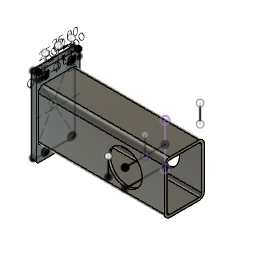
Ensamble-SC280 (Autodesk Fusion 360 archive; units mm, degrees)
design "ApoyoEje1" references "Chasis-V0"
Autodesk Fusion 360 part; units mm, degrees
ref_plane "WorkPlane1" through (506, 300, 480) normal (1, 0, 0) x (0, 1, 0)
sketch "Sketch1" plane through (506, 0, 0) normal (1, 0, 0) x (0, 1, 0)
  line L0 (260, 25) -> (340, 25)
  line L1 (340, 25) -> (340, 935)
  line L2 (340, 935) -> (260, 935)
  line L3 (260, 935) -> (260, 25)
  line L4 (0, 0) -> (600, 0) construction
  line L5 (0, 545) -> (600, 545) construction
  line L6 (328, 595) -> (272, 595)
  line L7 (262, 585) -> (262, 505)
  line L8 (272, 495) -> (328, 495)
  line L9 (338, 505) -> (338, 585)
  arc A0 (338, 585) -> (328, 595) centre (328, 585) ccw
  arc A1 (272, 595) -> (262, 585) centre (272, 585) ccw
  arc A2 (328, 495) -> (338, 505) centre (328, 505) ccw
  arc A3 (262, 505) -> (272, 495) centre (272, 505) ccw
  line L10 (272, 499.8) -> (328, 499.8)
  arc A4 (328, 499.8) -> (333.2, 505) centre (328, 505) ccw
  line L11 (333.2, 505) -> (333.2, 585)
  arc A5 (333.2, 585) -> (328, 590.2) centre (328, 585) ccw
  line L12 (328, 590.2) -> (272, 590.2)
  arc A6 (272, 590.2) -> (266.8, 585) centre (272, 585) ccw
  line L13 (266.8, 585) -> (266.8, 505)
  arc A7 (266.8, 505) -> (272, 499.8) centre (272, 505) ccw
  line L14 (300, 499.8) -> (300, 590.2) construction
  line L15 (333.2, 545) -> (266.8, 545) construction
  line L16 (258.75, 470) -> (341.25, 470)
  point P0 (262, 595)
  point P1 (262, 495)
  point P2 (338, 495)
  point P3 (300, 545)
  point P4 (300, 495)
  point P5 (262, 545)
  point P6 (300, 545)
  point P7 (300, 620)
  dimension "d1" = 76
  dimension "d2" = 100
  dimension "d3" = -4.8
  dimension "d5" = 300
  dimension "d6" = 10
  dimension "d7" = 10
  dimension "d8" = 10
  dimension "d9" = 10
  dimension "d11" = 300
  dimension "d12" = 545
  dimension "d35" = 82.5
  constraint coincident L4.start origin
  constraint horizontal L4
  constraint horizontal L5
  constraint horizontal L6
  constraint perpendicular L6 L7
  constraint parallel L6 L8
  constraint parallel L7 L9
  constraint midpoint L5 P6
  constraint tangent L6 A0
  constraint tangent L9 A0
  constraint coincident P0 L6
  constraint coincident P0 L7
  constraint tangent L6 A1
  constraint tangent L7 A1
  constraint coincident P2 L8
  constraint coincident P2 L9
  constraint tangent L8 A2
  constraint tangent L9 A2
  constraint coincident P1 L7
  constraint coincident P1 L8
  constraint tangent L7 A3
  constraint tangent L8 A3
  constraint midpoint L10 L14.start
  constraint midpoint L12 L14.end
  constraint midpoint L11 L15.start
  constraint midpoint L13 L15.end
  constraint midpoint L8 P4
  constraint midpoint L7 P5
  constraint coincident P6 P3
  measures "d1" distance of P1 P2
  measures "d2" distance of P0 P1
  measures "d5" horizontal distance of L4.start P6
  measures "d6" radius of A0
  measures "d7" radius of A1
  measures "d8" radius of A2
  measures "d9" radius of A3
  measures "d11" horizontal distance of L4.start P4
  measures "d12" vertical distance of L4.start P5
  measures "d35" distance of L16.start L16.end
extrude "Extrude1" add sketch "Sketch1" along normal blind 250 contours L6 L7 L8 L9 A0 A1 A2 A3 makes body 1
extrude "Extrude2" cut 1 faces at (506, 265.2, 558.3333) along direction (1, 0, 0) blind 9.5 on bodies 1 bodies 1
sketch "Sketch2" plane through (0, 262, 0) normal (0, -1, 0) x (1, 0, 0)
  line L0 (515.5, 585) -> (515.5, 505)
  line L1 (515.5, 505) -> (756, 505)
  line L2 (756, 505) -> (756, 585)
  line L3 (756, 585) -> (515.5, 585)
  line L4 (756, 545) -> (756, 700) construction
  line L5 (681, 545) -> (681, 700) construction
  circle A0 centre (681, 545) radius 32.5
  circle A1 centre (681, 545) radius 13
  circle A2 centre (681, 545) radius 26
  circle A3 centre (681, 545) radius 22.5
  dimension "d18" = -75
  dimension "d19" = 65
  dimension "d20" = 26
  dimension "d21" = 52
  dimension "d22" = 45
  constraint midpoint L2 L4.start
  constraint perpendicular L3 L4
  constraint coincident L5.start A0.centre
  constraint concentric A0 A1
  constraint concentric A0 A2
  constraint concentric A1 A3
  measures "d19" diameter of A0
  measures "d20" diameter of A1
  measures "d21" diameter of A2
  measures "d22" diameter of A3
extrude "Extrude6" cut sketch "Sketch2" against normal up to surface (76 mm away) contours A0 | A1 | A2 | A3 bodies 1
sketch "Sketch5" plane through (506, 300, 480) normal (1, 0, 0) x (0, 1, 0)
  line L0 (38.25, 140) -> (-38.25, 140)
  line L1 (-41.25, 137) -> (-41.25, -7)
  line L2 (-38.25, -10) -> (38.25, -10)
  line L3 (41.25, -7) -> (41.25, 137)
  line L4 (41.25, 140) -> (-41.25, -10) construction
  line L5 (-41.25, 140) -> (41.25, -10) construction
  arc A0 (41.25, 137) -> (38.25, 140) centre (38.25, 137) ccw
  arc A1 (-38.25, 140) -> (-41.25, 137) centre (-38.25, 137) ccw
  arc A2 (-41.25, -7) -> (-38.25, -10) centre (-38.25, -7) ccw
  arc A3 (38.25, -10) -> (41.25, -7) centre (38.25, -7) ccw
  point P0 (0, 65)
  dimension "d40" = 82.5
  dimension "d41" = 150
  dimension "d44" = 3
  dimension "d45" = 3
  dimension "d46" = 3
  dimension "d47" = 3
  constraint horizontal L0
  constraint perpendicular L0 L1
  constraint parallel L0 L2
  constraint parallel L1 L3
  constraint coincident L4 P0
  constraint coincident L5 P0
  constraint coincident L4.start L3
  constraint coincident L4.start L0
  constraint tangent L3 A0
  constraint tangent L0 A0
  constraint coincident L5.start L0
  constraint coincident L5.start L1
  constraint tangent L0 A1
  constraint tangent L1 A1
  constraint coincident L4.end L1
  constraint coincident L4.end L2
  constraint tangent L1 A2
  constraint tangent L2 A2
  constraint coincident L5.end L3
  constraint coincident L5.end L2
  constraint tangent L3 A3
  constraint tangent L2 A3
  measures "d40" distance of L4.end L5.end
  measures "d41" distance of L5.start L4.end
  measures "d44" radius of A0
  measures "d45" radius of A1
  measures "d46" radius of A2
  measures "d47" radius of A3
extrude "Extrude8" add sketch "Sketch5" along normal blind 9.5 separate body makes body 2
sketch "Sketch6" plane through (515.5, 0, 0) normal (1, 0, 0) x (0, 1, 0)
  arc A0 (338.25, 470) -> (341.25, 473) centre (338.25, 473) ccw
  line L0 (341.25, 473) -> (341.25, 617)
  arc A1 (341.25, 617) -> (338.25, 620) centre (338.25, 617) ccw
  line L1 (338.25, 620) -> (261.75, 620)
  arc A2 (261.75, 620) -> (258.75, 617) centre (261.75, 617) ccw
  line L2 (258.75, 617) -> (258.75, 473)
  arc A3 (258.75, 473) -> (261.75, 470) centre (261.75, 473) ccw
  line L3 (261.75, 470) -> (338.25, 470)
  line L4 (261.75, 620) -> (338.25, 620) construction
  line L5 (261.75, 608) -> (338.25, 608) construction
  line L6 (300, 608) -> (300, 645) construction
  line L7 (325, 608) -> (325, 645) construction
  line L8 (275, 608) -> (275, 645) construction
  circle A4 centre (275, 608) radius 6.5
  circle A5 centre (325, 608) radius 6.5
  line L9 (341.25, 545) -> (258.75, 545) construction
  circle A6 centre (325, 482) radius 6.5
  circle A7 centre (275, 482) radius 6.5
  dimension "d48" = 12
  dimension "d49" = 25
  dimension "d50" = -25
  dimension "d51" = 13
  dimension "d52" = 13
  constraint coincident L1.end A2.start
  constraint coincident A1.end L1.start
  constraint midpoint L5 L6.start
  constraint perpendicular L5 L6
  constraint coincident L8.start A4.centre
  constraint coincident L7.start A5.centre
  constraint midpoint L0 L9.start
  constraint midpoint L2 L9.end
  constraint symmetric A4 L9 A7
  constraint symmetric A5 L9 A6
  measures "d51" diameter of A4
  measures "d52" diameter of A5
ref_plane "WorkPlane2" through (681, 300, 545) normal (1, 0, 0) x (0, 1, 0)
sketch "Sketch8" plane through (681, 300, 545) normal (1, 0, 0) x (0, 1, 0)
  line L0 (38, -40) -> (38, 40)
  line L1 (-38, 0) -> (38, 0)
  line L2 (0, 0) -> (0, 34.845)
  line L3 (-70, 0) -> (-70, 34.845)
  line L4 (105, 0) -> (105, 34.845)
  line L5 (-38, -35) -> (38, -35)
  point P0 (-38, 0)
  point P1 (38, 0)
  dimension "d56" = -70
  dimension "d57" = 105
  dimension "d58" = 35
  constraint coincident P0 L1.start
  constraint coincident P1 L1.end
  constraint coincident L2.start origin
  constraint perpendicular L1 L2
extrude "Extrude9" [suppressed]
sketch "Sketch7" plane through (506, 0, 0) normal (1, 0, 0) x (0, 1, 0)

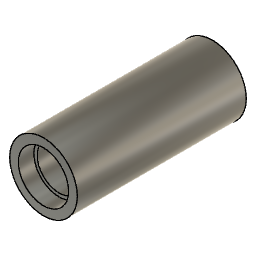
design "CamisaEje"
Autodesk Fusion 360 part; units mm, degrees
sketch "Sketch1" plane through (0, 0, 0) normal (0, 1, 0) x (1, 0, 0)
  circle A0 centre (0, 0) radius 35
  circle A1 centre (0, 0) radius 22.5
  dimension "d1" = 70
  dimension "d3" = 45
  constraint coincident A0.centre A1.centre
  measures "d1" diameter of A0
  measures "d3" diameter of A1
extrude "Extrude1" add sketch "Sketch1" along normal blind 140 and the other way blind 35
sketch "Sketch2" plane through (0, -35, 0) normal (0, -1, 0) x (1, 0, 0)
  circle A0 centre (0, 0) radius 22.5
  circle A1 centre (0, 0) radius 35
  circle A2 centre (0, 0) radius 26
  dimension "d8" = 52
  constraint coincident A0.centre A1.centre
  measures "d8" diameter of A2
extrude "Extrude2" cut sketch "Sketch2" against normal blind 16 contours A2
sketch "Sketch3" plane through (0, 140, 0) normal (0, 1, 0) x (-1, 0, 0)
  circle A0 centre (0, 0) radius 22.5
  circle A1 centre (0, 0) radius 35
  circle A2 centre (0, 0) radius 26
  dimension "d11" = 52
  constraint coincident A0.centre A1.centre
  measures "d11" diameter of A2
extrude "Extrude3" cut sketch "Sketch3" against normal blind 16 contours A2

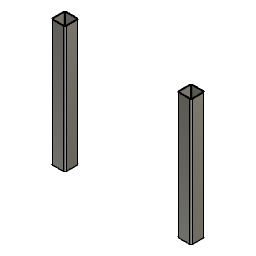
design "Chasis-V0"
Autodesk Fusion 360 part; units mm, degrees
sketch "Sketch1" plane through (0, 0, 0) normal (0, 0, 1) x (1, 0, 0)
  line L0 (0, 0) -> (0, 1000) construction
  line L1 (406, 0) -> (406, 1000) construction
  line L2 (-406, 0) -> (-406, 1000) construction
  line L3 (-406, 260) -> (-406, 340)
  line L4 (-416, 350) -> (-496, 350)
  line L5 (-506, 340) -> (-506, 260)
  line L6 (-496, 250) -> (-416, 250)
  line L7 (406, 0) -> (-406, 0) construction
  line L8 (406, 250) -> (-406, 250) construction
  arc A0 (-496, 350) -> (-506, 340) centre (-496, 340) ccw
  arc A1 (-406, 340) -> (-416, 350) centre (-416, 340) ccw
  arc A2 (-416, 250) -> (-406, 260) centre (-416, 260) ccw
  arc A3 (-506, 260) -> (-496, 250) centre (-496, 260) ccw
  line L9 (-410.8, 260) -> (-410.8, 340)
  arc A4 (-410.8, 340) -> (-416, 345.2) centre (-416, 340) ccw
  line L10 (-416, 345.2) -> (-496, 345.2)
  arc A5 (-496, 345.2) -> (-501.2, 340) centre (-496, 340) ccw
  line L11 (-501.2, 340) -> (-501.2, 260)
  arc A6 (-501.2, 260) -> (-496, 254.8) centre (-496, 260) ccw
  line L12 (-496, 254.8) -> (-416, 254.8)
  arc A7 (-416, 254.8) -> (-410.8, 260) centre (-416, 260) ccw
  point P0 (-406, 250)
  point P1 (-406, 350)
  point P2 (-506, 250)
  dimension "d3" = 100
  dimension "d4" = 100
  dimension "d7" = 10
  dimension "d8" = 10
  dimension "d9" = 10
  dimension "d10" = 10
  constraint coincident L0.start origin
  constraint perpendicular L2 L7
  constraint coincident P0 L8.end
  constraint tangent L5 A0
  constraint tangent L4 A0
  constraint coincident P1 L3
  constraint coincident P1 L4
  constraint tangent L3 A1
  constraint tangent L4 A1
  constraint coincident P0 L3
  constraint coincident P0 L6
  constraint tangent L3 A2
  constraint tangent L6 A2
  constraint coincident P2 L5
  constraint coincident P2 L6
  constraint tangent L5 A3
  constraint tangent L6 A3
  constraint parallel L0 L1
  constraint parallel L0 L2
  constraint parallel L3 L9
  constraint concentric A1 A4
  constraint parallel L4 L10
  constraint concentric A0 A5
  constraint parallel L5 L11
  constraint concentric A3 A6
  constraint parallel L6 L12
  constraint concentric A2 A7
  constraint tangent L9 A4
  constraint tangent L9 A7
  constraint tangent L11 A6
  constraint tangent L10 A5
  constraint tangent A4 L10
  constraint tangent A5 L11
  constraint tangent A6 L12
  constraint tangent L12 A7
  constraint parallel L7 L8
  measures "d3" distance of P0 P1
  measures "d4" distance of P0 P2
  measures "d7" radius of A0
  measures "d8" radius of A1
  measures "d9" radius of A2
  measures "d10" radius of A3
extrude "Extrude1" add sketch "Sketch1" along normal blind 935 makes body 1
extrude "Extrude2" cut 1 faces at (-409.2, 286.6667, 0) along direction (0, 0, 1) blind 25 on bodies 1 bodies 1
copy_body "CopyPasteBodies1" bodies 1 makes body 2
move_body "Move1" bodies 2 to x (1, 0, 0) y (0, 1, 0) z (0, 0, 1) at (912, 0, 0)

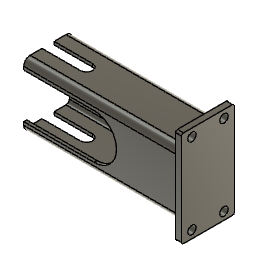
design "ApoyoEje2"
Autodesk Fusion 360 part; units mm, degrees
ref_plane "WorkPlane1" through (-515.5, 300, 480) normal (-1, 0, 0) x (0, -1, 0)
sketch "Sketch1" plane through (-515.5, 300, 480) normal (-1, 0, 0) x (0, 1, 0)
sketch "Sketch2" plane through (-515.5, 300, 480) normal (-1, 0, 0) x (0, 1, 0)
  arc A0 (-28, -19.8) -> (-33.2, -25) centre (-28, -25) ccw
  line L0 (-41.25, -140) -> (41.25, -140)
  arc A1 (33.2, -25) -> (28, -19.8) centre (28, -25) ccw
  line L1 (33.2, -65) -> (-33.2, -65) construction
  line L2 (-38, -25) -> (-38, -105)
  arc A2 (-28, -15) -> (-38, -25) centre (-28, -25) ccw
  arc A3 (38, -25) -> (28, -15) centre (28, -25) ccw
  arc A4 (-33.2, -105) -> (-28, -110.2) centre (-28, -105) ccw
  arc A5 (28, -110.2) -> (33.2, -105) centre (28, -105) ccw
  line L3 (-28, -115) -> (28, -115)
  line L4 (33.2, -105) -> (33.2, -25)
  line L5 (38, -105) -> (38, -25)
  line L6 (28, -19.8) -> (-28, -19.8)
  line L7 (-28, -110.2) -> (28, -110.2)
  line L8 (-33.2, -25) -> (-33.2, -105)
  arc A6 (-38, -105) -> (-28, -115) centre (-28, -105) ccw
  line L9 (28, -15) -> (-28, -15)
  arc A7 (28, -115) -> (38, -105) centre (28, -105) ccw
  line L10 (0, -110.2) -> (0, -19.8) construction
  line L11 (40, 455) -> (-40, 455)
  point P0 (38, -115)
  point P1 (0, -65)
  point P2 (-38, -15)
  point P3 (-38, -115)
  point P4 (-38, -65)
  point P5 (0, -115)
  point P6 (0, 10)
  point P7 (0, -65)
  dimension "d3" = -4.8
  dimension "d4" = 76
  dimension "d5" = 100
  dimension "d6" = 10
  dimension "d7" = 10
  dimension "d8" = 10
  dimension "d9" = 10
  dimension "d35" = 82.5
  dimension "d12" = 570
  dimension "d13" = 38
  constraint horizontal L9
  constraint perpendicular L2 L9
  constraint parallel L3 L9
  constraint parallel L2 L5
  constraint tangent A3 L9
  constraint tangent A3 L5
  constraint coincident P2 L9
  constraint coincident P2 L2
  constraint tangent A2 L9
  constraint tangent L2 A2
  constraint coincident P0 L3
  constraint coincident P0 L5
  constraint tangent L3 A7
  constraint tangent L5 A7
  constraint coincident P3 L2
  constraint coincident P3 L3
  constraint tangent L2 A6
  constraint tangent L3 A6
  constraint midpoint L10.start L7
  constraint midpoint L10.end L6
  constraint midpoint L1.start L4
  constraint midpoint L1.end L8
  constraint midpoint P5 L3
  constraint midpoint P4 L2
  constraint coincident P7 P1
  measures "d4" distance of P0 P3
  measures "d5" distance of P2 P3
  measures "d6" radius of A3
  measures "d7" radius of A2
  measures "d8" radius of A7
  measures "d9" radius of A6
  measures "d35" distance of L0.start L0.end
  measures "d12" distance of L3 L11
  measures "d13" distance of origin L5
extrude "Extrude1" add sketch "Sketch2" along normal blind 240.5
ref_plane "WorkPlane2" through (-506, 300, 480) normal (-1, 0, 0) x (0, -1, 0)
sketch "Sketch3" plane through (0, 262, 0) normal (0, -1, 0) x (1, 0, 0)
  line L0 (-515.5, 505) -> (-515.5, 585)
  line L1 (-515.5, 585) -> (-756, 585)
  line L2 (-756, 585) -> (-756, 505) construction
  line L3 (-756, 505) -> (-515.5, 505)
  line L4 (-646, 585) -> (-646, 505)
  line L5 (-646, 510) -> (-756, 510)
  line L6 (-646, 580) -> (-756, 580)
  arc A0 (-646, 510) -> (-646, 580) centre (-646, 545) ccw
  line L7 (-756, 510) -> (-756, 580)
  dimension "d20" = -110
  dimension "d21" = 70
  constraint midpoint L4 A0.centre
  constraint coincident L4 L5.start
  constraint coincident L2 L5.end
  constraint tangent L5 A0
  constraint coincident L4 L6.start
  constraint coincident L2 L6.end
  constraint tangent L6 A0
  measures "d21" diameter of A0
extrude "Extrude2" cut sketch "Sketch3" against normal up to surface (76 mm away) contours L4 L5 L6 L7 | L4 A0
sketch "Sketch4" plane through (0, 0, 595) normal (0, 0, 1) x (-1, 0, 0)
  line L0 (515.5, -272) -> (515.5, -328)
  line L1 (515.5, -328) -> (756, -328)
  line L2 (756, -328) -> (756, -272) construction
  line L3 (756, -272) -> (515.5, -272)
  line L4 (696, -328) -> (696, -272)
  line L5 (696, -290.5) -> (756, -290.5)
  line L6 (696, -309.5) -> (756, -309.5)
  arc A0 (696, -290.5) -> (696, -309.5) centre (696, -300) ccw
  line L7 (756, -290.5) -> (756, -309.5)
  dimension "d24" = -60
  dimension "d25" = 19
  constraint midpoint L4 A0.centre
  constraint coincident L4 L5.start
  constraint coincident L2 L5.end
  constraint tangent L5 A0
  constraint coincident L4 L6.start
  constraint coincident L2 L6.end
  constraint tangent L6 A0
  measures "d25" diameter of A0
extrude "Extrude3" cut sketch "Sketch4" against normal up to surface (100 mm away) contours L4 L5 L6 L7 | L4 A0
sketch "Sketch5" plane through (-506, 300, 480) normal (-1, 0, 0) x (0, 1, 0)
  arc A0 (38.25, -140) -> (41.25, -137) centre (38.25, -137) ccw
  line L0 (-38.25, -140) -> (38.25, -140)
  circle A1 centre (25, -128) radius 6.5
  circle A2 centre (-25, -128) radius 6.5
  arc A3 (-41.25, -137) -> (-38.25, -140) centre (-38.25, -137) ccw
  line L1 (-41.25, 7) -> (-41.25, -137)
  line L2 (41.25, -137) -> (41.25, 7)
  arc A4 (-38.25, 10) -> (-41.25, 7) centre (-38.25, 7) ccw
  line L3 (38.25, 10) -> (-38.25, 10)
  arc A5 (41.25, 7) -> (38.25, 10) centre (38.25, 7) ccw
  line L4 (-38.25, 10) -> (38.25, 10) construction
  line L5 (-38.25, -2) -> (38.25, -2) construction
  circle A6 centre (25, -2) radius 6.5
  circle A7 centre (-25, -2) radius 6.5
  line L6 (-41.25, -65) -> (41.25, -65) construction
  line L7 (33.2, -65) -> (-33.2, -65)
  point P0 (25, -2)
  point P1 (0, -2)
  point P2 (-25, -2)
  dimension "d48" = 12
  dimension "d51" = 13
  dimension "d52" = 13
  constraint coincident A4.start L3.end
  constraint coincident L3.start A5.end
  constraint midpoint P1 L5
  constraint coincident P2 A7.centre
  constraint coincident P0 A6.centre
  constraint midpoint L1 L6.start
  constraint midpoint L2 L6.end
  constraint perpendicular L2 L6
  measures "d51" diameter of A7
  measures "d52" diameter of A6
extrude "Extrude4" add sketch "Sketch5" along normal blind 9.5

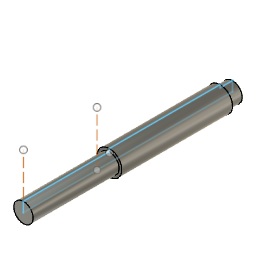
design "EjeVolante"
Autodesk Fusion 360 part; units mm, degrees
sketch "Sketch2" plane through (0, 0, 0) normal (1, 0, 0) x (0, 1, 0)
  line L0 (-35, 0) -> (-35, 70) construction
  line L1 (-130, 0) -> (-130, 70) construction
  line L2 (-130, 0) -> (140, 0) construction
  line L3 (-19, 16) -> (-19, 11)
  line L4 (-19, 16) -> (124, 16)
  line L5 (124, 16) -> (124, 12.5)
  line L6 (-130, 12.5) -> (-19, 12.5)
  line L7 (124, 12.5) -> (140, 12.5)
  line L8 (140, 0) -> (140, 12.5)
  line L9 (-130, 0) -> (-130, 12.5)
  line L10 (-130, 0) -> (140, 0)
  dimension "d1" = -95
  constraint vertical L0
  constraint perpendicular L1 L2
  constraint perpendicular L2 L5
  constraint perpendicular L3 L6
  constraint coincident L5.end L6
  constraint parallel L2 L6
  constraint coincident L3 L6.end
  constraint perpendicular L2 L8
  constraint perpendicular L2 L9
revolve "Revolve1" add sketch "Sketch2" angle 360 about axis through (0, -130, 0) along (0, 1, 0)
